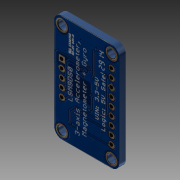
# Autodesk Inventor part: Adafruit Compass
Saved by Autodesk Inventor 2015 (Build 190159000, 159)
## iProperties
Created: 2015-11-02
Part Number: Adafruit Compass
Material: Generic
Document SubType Name: Modeling
Designer: James
Density: 1 g/cm^3
Appearance: Default
Author: James
Autodesk Inventor part; units mm, degrees
ref_plane "YZ Plane" through (0, 0, 0) normal (1, 0, 0) x (0, 1, 0)
ref_plane "XZ Plane" through (0, 0, 0) normal (0, 1, 0) x (-1, 0, 0)
ref_plane "XY Plane" through (0, 0, 0) normal (0, 0, 1) x (1, 0, 0)
sketch "Sketch1" plane through (0, 0, 0) normal (0, 1, 0) x (-1, 0, 0)
  line L0 (-10, 14) -> (-10, -14)
  line L1 (-7.5, -16.5) -> (7.5, -16.5)
  line L2 (10, -14) -> (10, 14)
  line L3 (7.5, 16.5) -> (-7.5, 16.5)
  line L4 (-10, 16.5) -> (10, -16.5) construction
  line L5 (-10, -16.5) -> (10, 16.5) construction
  arc A0 (10, 14) -> (7.5, 16.5) centre (7.5, 14) ccw
  arc A1 (7.5, -16.5) -> (10, -14) centre (7.5, -14) ccw
  arc A2 (-10, -14) -> (-7.5, -16.5) centre (-7.5, -14) ccw
  arc A3 (-7.5, 16.5) -> (-10, 14) centre (-7.5, 14) ccw
  circle A4 centre (7.5, 14) radius 1.25
  circle A5 centre (-7.5, 14) radius 1.25
  circle A6 centre (-7.5, -14) radius 1.25
  circle A7 centre (7.5, -14) radius 1.25
  point P0 (0, 0)
  dimension "d0" = 33
  dimension "d1" = 20
  dimension "d2" = 2.5
  dimension "d3" = 2.5
  dimension "d4" = 2.5
  dimension "d5" = 2.5
  dimension "d6" = 2.5
  constraints: 12 end point, 8 centre point, 8 point on circle, 8 point on line, 8 tangent, 4 coincident, 3 equal radius, 2 midpoint, 2 parallel, 1 perpendicular, 1 vertical
  measures "d0" distance of L4.start L5.start
  measures "d1" distance of L4.end L5.start
  measures "d2" radius of A0
  measures "d3" diameter of A4
  measures "d4" diameter of A5
  measures "d5" diameter of A6
  measures "d6" diameter of A7
extrude "Extrusion1" add sketch "Sketch1" along normal blind 2
sketch "Sketch2" plane through (0, 2, 0) normal (0, 1, 0) x (1, 0, 0)
  line L0 (-17.9692, -32.7187) -> (-17.5216, 33.3599) construction
  line L1 (-17.5216, 33.3599) -> (32.0714, 33.0239) construction
  line L2 (32.0714, 33.0239) -> (31.6238, -33.0546) construction
  line L3 (31.6238, -33.0546) -> (-17.9692, -32.7187) construction
  circle A0 centre (-7.5, 14) radius 1.25 projected
  circle A1 centre (7.5, 14) radius 1.25 projected
  circle A2 centre (7.5, -14) radius 1.25 projected
  circle A3 centre (-7.5, -14) radius 1.25 projected
  line L4 (-10, 14) -> (-10, -14) projected
  arc A4 (-10, -14) -> (-7.5, -16.5) centre (-7.5, -14) ccw projected
  line L5 (-7.5, -16.5) -> (7.5, -16.5) projected
  arc A5 (7.5, -16.5) -> (10, -14) centre (7.5, -14) ccw projected
  line L6 (10, -14) -> (10, 14) projected
  arc A6 (10, 14) -> (7.5, 16.5) centre (7.5, 14) ccw projected
  line L7 (7.5, 16.5) -> (-7.5, 16.5) projected
  arc A7 (-7.5, 16.5) -> (-10, 14) centre (-7.5, 14) ccw projected
  point P0 (0, 0)
  constraints: 2 other
decal "Decal1"
sketch "Sketch3" plane through (0, 0, 0) normal (0, -1, 0) x (1, 0, 0)
  circle A0 centre (-7.5, -14) radius 1.25 projected
  circle A1 centre (7.5, -14) radius 1.25 projected
  circle A2 centre (7.5, 14) radius 1.25 projected
  circle A3 centre (-7.5, 14) radius 1.25 projected
  line L0 (-10, 14) -> (-10, -14) projected
  arc A4 (-10, -14) -> (-7.5, -16.5) centre (-7.5, -14) ccw projected
  line L1 (-7.5, -16.5) -> (7.5, -16.5) projected
  arc A5 (7.5, -16.5) -> (10, -14) centre (7.5, -14) ccw projected
  line L2 (10, -14) -> (10, 14) projected
  arc A6 (10, 14) -> (7.5, 16.5) centre (7.5, 14) ccw projected
  line L3 (7.5, 16.5) -> (-7.5, 16.5) projected
  arc A7 (-7.5, 16.5) -> (-10, 14) centre (-7.5, 14) ccw projected
  line L4 (-25.6164, -20.5771) -> (-25.6164, 49.1548) construction
  line L5 (-25.6164, 49.1548) -> (26.7185, 49.1548) construction
  line L6 (26.7185, 49.1548) -> (26.7185, -20.5771) construction
  line L7 (26.7185, -20.5771) -> (-25.6164, -20.5771) construction
  line L8 (-7.5, 16.5) -> (7.5, 16.5) projected
  line L9 (0, 16.5) -> (0, 0)
  constraints: 2 end point, 1 midpoint, 1 vertical, 2 other
decal "Decal2"
body "Solid1"
